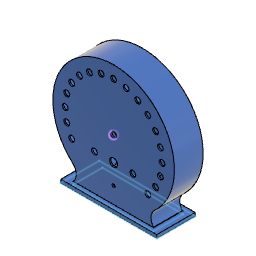
Minutka (Autodesk Fusion 360 design; units mm, degrees)
Autodesk Fusion 360 part; units mm, degrees
sketch "Sketch1" plane through (0, 0, 0) normal (0, 1, 0) x (1, 0, 0)
  circle A0 centre (0, 0) radius 35.5
  circle A1 centre (0, 0) radius 37
  circle A2 centre (0, 0) radius 38
  line L0 (-25, 37.5) -> (25, 37.5)
  line L1 (25, 37.5) -> (25, 39.5)
  line L2 (25, 39.5) -> (-25, 39.5)
  line L3 (-25, 39.5) -> (-25, 37.5)
  arc A3 (-25.5469, 28.131) -> (-25, 37.5) centre (-30.0546, 33.0946) ccw
  arc A4 (25, 37.5) -> (25.5469, 28.131) centre (30.0546, 33.0946) ccw
  dimension "d1" = 71
  dimension "d2" = 74
  dimension "d3" = 76
  dimension "d4" = 50
  dimension "d5" = 2
  dimension "d6" = 37.5
  dimension "d7" = 25
  constraint coincident A0.centre A1.centre
  constraint concentric A1 A2
  constraint horizontal L0
  constraint vertical L1
  constraint horizontal L2
  constraint vertical L3
  constraint tangent A2 A3
  constraint coincident A2 A3.start
  measures "d1" diameter of A0
  measures "d2" diameter of A1
  measures "d3" diameter of A2
  measures "d4" distance of L0.start L0.end
  measures "d5" distance of L0.start L2.end
  measures "d6" vertical distance of A0.centre L0.end
  measures "d7" horizontal distance of A0.centre L0.end
extrude "Extrude1" add sketch "Sketch1" along normal blind 18 contours A2 L0 | A2 L0 A4 | A2 L0 A3 | A2 L0 | A2 L0 L1 L2 L3 makes body 1
extrude "Extrude2" add sketch "Sketch1" along normal blind 17.2 contours A1 bodies 1
extrude "Extrude3" add sketch "Sketch1" along normal blind 0.8 contours A0 bodies 1
sketch "Sketch2" plane through (0, 17.2, 0) normal (0, 1, 0) x (-1, 0, 0)
  circle A0 centre (0, 0) radius 35.5
  circle A1 centre (0, 0) radius 37
  line L0 (-1.5, 38.5) -> (1.5, 38.5)
  line L1 (1.5, 38.5) -> (1.5, 35)
  line L2 (1.5, 35) -> (-1.5, 35)
  line L3 (-1.5, 35) -> (-1.5, 38.5)
  line L4 (-1.5, -42.5) -> (1.5, -42.5)
  line L5 (1.5, -42.5) -> (1.5, -34.5)
  line L6 (1.5, -34.5) -> (-1.5, -34.5)
  line L7 (-1.5, -34.5) -> (-1.5, -42.5)
  constraint horizontal L0
  constraint vertical L1
  constraint horizontal L2
  constraint vertical L3
  constraint horizontal L4
  constraint vertical L5
  constraint horizontal L6
  constraint vertical L7
extrude "Extrude4" cut sketch "Sketch2" against normal blind 1 contours A0 A1 L1 L3 | A0 A1 L5 L7 bodies 1
sketch "Sketch3" plane through (0, 0, 0) normal (0, 1, 0) x (1, 0, 0)
  circle A0 centre (-30.3, 0) radius 1.8
  circle A1 centre (-29.2676, 7.8422) radius 1.8
  circle A2 centre (-26.2406, 15.15) radius 1.8
  circle A3 centre (-29.2676, -7.8422) radius 1.8
  circle A4 centre (-26.2406, -15.15) radius 1.8
  circle A5 centre (-21.4253, -21.4253) radius 1.8
  circle A6 centre (-15.15, -26.2406) radius 1.8
  circle A7 centre (-7.8422, -29.2676) radius 1.8
  circle A8 centre (0, -30.3) radius 1.8
  circle A9 centre (7.8422, -29.2676) radius 1.8
  circle A10 centre (15.15, -26.2406) radius 1.8
  circle A11 centre (21.4253, -21.4253) radius 1.8
  circle A12 centre (26.2406, -15.15) radius 1.8
  circle A13 centre (29.2676, -7.8422) radius 1.8
  circle A14 centre (30.3, 0) radius 1.8
  circle A15 centre (29.2676, 7.8422) radius 1.8
  circle A16 centre (26.2406, 15.15) radius 1.8
  circle A17 centre (21.4253, 21.4253) radius 1.8
  circle A18 centre (0, 0) radius 1.8
  circle A19 centre (0, 27.5) radius 1
  circle A20 centre (0, 15) radius 2.5
  circle A21 centre (-12, 15) radius 1.8
  circle A22 centre (12, 15) radius 1.8
  dimension "d16" = 3.6
  dimension "d17" = 30.3
  dimension "d19" = -30
  dimension "d21" = 225
  dimension "d22" = 3.6
  dimension "d23" = 2
  dimension "d24" = 27.5
  dimension "d25" = 5
  dimension "d26" = 15
  dimension "d27" = 3.6
  dimension "d28" = 12
  dimension "d29" = 3.6
  dimension "d30" = 12
  constraint coincident A18.centre origin
  measures "d16" diameter of A0
  measures "d17" distance of A18.centre A0.centre
  measures "d22" diameter of A18
  measures "d23" diameter of A19
  measures "d24" distance of A18.centre A19.centre
  measures "d25" diameter of A20
  measures "d26" distance of A18.centre A20.centre
  measures "d27" diameter of A21
  measures "d28" distance of A20.centre A21.centre
  measures "d29" diameter of A22
  measures "d30" distance of A20.centre A22.centre
extrude "Extrude5" cut sketch "Sketch3" along normal blind 0.8 bodies 1
sketch "Sketch4" plane through (0, 0, 0) normal (0, -1, 0) x (1, 0, 0)
  circle A0 centre (12, -15) radius 1.8
  circle A1 centre (26.2406, -15.15) radius 1.8
  circle A2 centre (26.2406, 15.15) radius 1.8
  circle A3 centre (0, 30.3) radius 1.8
  circle A4 centre (-26.2406, 15.15) radius 1.8
  circle A5 centre (-26.2406, -15.15) radius 1.8
  circle A6 centre (-29.2676, 7.8422) radius 1.8
  circle A7 centre (-7.8422, 29.2676) radius 1.8
  circle A8 centre (21.4253, 21.4253) radius 1.8
  circle A9 centre (29.2676, -7.8422) radius 1.8
  circle A10 centre (0, -15) radius 2.5
  circle A11 centre (-12, -15) radius 1.8
  circle A12 centre (21.4253, -21.4253) radius 1.8
  circle A13 centre (29.2676, 7.8422) radius 1.8
  circle A14 centre (7.8422, 29.2676) radius 1.8
  circle A15 centre (-21.4253, 21.4253) radius 1.8
  circle A16 centre (-29.2676, -7.8422) radius 1.8
  circle A17 centre (-30.3, 0) radius 1.8
  circle A18 centre (-15.15, 26.2406) radius 1.8
  circle A19 centre (15.15, 26.2406) radius 1.8
  circle A20 centre (30.3, 0) radius 1.8
  circle A21 centre (0, -27.5) radius 1
  circle A22 centre (0, 0) radius 1.8
  line L0 (-25, -39.5) -> (25, -39.5)
  line L1 (25, -39.5) -> (25, -37.5)
  arc A23 (25.5469, -28.131) -> (25, -37.5) centre (30.0546, -33.0946) ccw
  arc A24 (25.5469, -28.131) -> (-25.5469, -28.131) centre (0, 0) ccw
  arc A25 (-25, -37.5) -> (-25.5469, -28.131) centre (-30.0546, -33.0946) ccw
  line L2 (-25, -37.5) -> (-25, -39.5)
  circle A26 centre (-10, -22.5) radius 3
  circle A27 centre (10, -22.5) radius 3
  circle A28 centre (0, 23) radius 3
  circle A29 centre (8, 23) radius 3
  dimension "d33" = 6
  dimension "d34" = 22.5
  dimension "d35" = 10
  dimension "d36" = 6
  dimension "d37" = 10
  dimension "d38" = 22.5
  dimension "d39" = 6
  dimension "d40" = 23
  dimension "d41" = 6
  dimension "d42" = 8
  measures "d33" diameter of A26
  measures "d34" vertical distance of A22.centre A26.centre
  measures "d35" horizontal distance of A22.centre A26.centre
  measures "d36" diameter of A27
  measures "d37" horizontal distance of A22.centre A27.centre
  measures "d38" vertical distance of A22.centre A27.centre
  measures "d39" diameter of A28
  measures "d40" distance of A22.centre A28.centre
  measures "d41" diameter of A29
  measures "d42" distance of A28.centre A29.centre
extrude "Extrude6" add sketch "Sketch4" against normal blind 8.8 contours A26 | A29 bodies 1
extrude "Extrude7" add sketch "Sketch4" against normal blind 17.2 contours A27 | A28 bodies 1
sketch "Sketch5" plane through (0, 8.8, 0) normal (0, 1, 0) x (-1, 0, 0)
  circle A0 centre (-8, 23) radius 3
  circle A1 centre (-8, 23) radius 1.25
  circle A2 centre (10, -22.5) radius 1.25
  dimension "d47" = 2.5
  dimension "d48" = 2.5
  constraint concentric A0 A1
  measures "d47" diameter of A1
  measures "d48" diameter of A2
extrude "Extrude8" cut sketch "Sketch5" against normal blind 7 contours A1 | A2 bodies 1
sketch "Sketch6" plane through (0, 17.2, 0) normal (0, 1, 0) x (-1, 0, 0)
  circle A0 centre (0, 23) radius 3
  circle A1 centre (0, 23) radius 1.25
  circle A2 centre (-10, -22.5) radius 1.25
  dimension "d51" = 2.5
  dimension "d52" = 2.5
  constraint concentric A0 A1
  measures "d51" diameter of A1
  measures "d52" diameter of A2
sketch "Sketch7" plane through (0, 0.8, 0) normal (0, 1, 0) x (-1, 0, 0)
  circle A0 centre (-10, -22.5) radius 3
  circle A1 centre (0, 23) radius 3
  circle A2 centre (10, -22.5) radius 3
  circle A3 centre (-8, 23) radius 3
  circle A4 centre (-12, -15) radius 1.8
  circle A5 centre (-26.2406, -15.15) radius 1.8
  circle A6 centre (-26.2406, 15.15) radius 1.8
  circle A7 centre (0, 30.3) radius 1.8
  circle A8 centre (26.2406, 15.15) radius 1.8
  circle A9 centre (26.2406, -15.15) radius 1.8
  circle A10 centre (29.2676, 7.8422) radius 1.8
  circle A11 centre (7.8422, 29.2676) radius 1.8
  circle A12 centre (-21.4253, 21.4253) radius 1.8
  circle A13 centre (-29.2676, -7.8422) radius 1.8
  circle A14 centre (0, -15) radius 2.5
  circle A15 centre (12, -15) radius 1.8
  circle A16 centre (-21.4253, -21.4253) radius 1.8
  circle A17 centre (-29.2676, 7.8422) radius 1.8
  circle A18 centre (-7.8422, 29.2676) radius 1.8
  circle A19 centre (21.4253, 21.4253) radius 1.8
  circle A20 centre (29.2676, -7.8422) radius 1.8
  circle A21 centre (30.3, 0) radius 1.8
  circle A22 centre (15.15, 26.2406) radius 1.8
  circle A23 centre (-15.15, 26.2406) radius 1.8
  circle A24 centre (-30.3, 0) radius 1.8
  circle A25 centre (0, -27.5) radius 1
  circle A26 centre (0, 0) radius 1.8
  circle A27 centre (0, 0) radius 35.5
extrude "Extrude9" cut sketch "Sketch6" against normal blind 12 contours A1 | A2 bodies 1
sketch "Sketch8" plane through (0, 17.2, 0) normal (0, 1, 0) x (-1, 0, 0)
  line L0 (-1.5, 35.4683) -> (-1.5, 36.9696)
  arc A0 (-1.5, 36.9696) -> (-1.5, -36.9696) centre (0, 0) ccw
  line L1 (-1.5, -36.9696) -> (-1.5, -35.4683)
  arc A1 (-1.5, 35.4683) -> (-1.5, -35.4683) centre (0, 0) ccw
  circle A2 centre (0, 0) radius 36.5
  line L2 (-1.25, 38.5) -> (1.25, 38.5)
  line L3 (1.25, 38.5) -> (1.25, 34.7673)
  line L4 (1.25, 34.7673) -> (-1.25, 34.7673)
  line L5 (-1.25, 34.7673) -> (-1.25, 38.5)
  circle A3 centre (0, 0) radius 37
  line L6 (-1.25, -34) -> (1.25, -34)
  line L7 (1.25, -34) -> (1.25, -38.157)
  line L8 (1.25, -38.157) -> (-1.25, -38.157)
  line L9 (-1.25, -38.157) -> (-1.25, -34)
  circle A4 centre (-10, -22.5) radius 1.5
  circle A5 centre (0, 23) radius 1.5
  dimension "d55" = 73
  dimension "d56" = 2.5
  dimension "d57" = 1.25
  dimension "d58" = 2.5
  dimension "d59" = 1.25
  dimension "d60" = 3
  dimension "d61" = 3
  constraint coincident A0.centre A1.centre
  constraint horizontal L2
  constraint vertical L3
  constraint horizontal L4
  constraint vertical L5
  constraint horizontal L6
  constraint vertical L7
  constraint horizontal L8
  constraint vertical L9
  measures "d55" diameter of A2
  measures "d56" distance of L2.start L2.end
  measures "d57" horizontal distance of L2.start A0.centre
  measures "d58" distance of L6.start L6.end
  measures "d59" horizontal distance of A0.centre L6.start
  measures "d60" diameter of A4
  measures "d61" diameter of A5
extrude "Extrude10" add sketch "Sketch8" along normal blind 0.8 separate body contours L0 L1 A1 A2 | L0 L1 A1 A2 L3 L4 L5 L6 L7 L9 | A2 L3 L4 L5 | A2 L6 L7 L9 makes body 2
extrude "Extrude11" add sketch "Sketch8" against normal blind 0.5 contours A2 L3 L4 L5 | A2 L6 L7 L9 bodies 2
sketch "Sketch9" plane through (0, 0, 0) normal (0, 0, 1) x (1, 0, 0)
  line L0 (-30, 21, -39.5) -> (30, 21, -39.5)
  line L1 (30, 21, -39.5) -> (30, -3, -39.5)
  line L2 (30, -3, -39.5) -> (-30, -3, -39.5)
  line L3 (-30, -3, -39.5) -> (-30, 21, -39.5)
  line L4 (-25.25, 18.25, -39.5) -> (25.25, 18.25, -39.5)
  line L5 (25.25, 18.25, -39.5) -> (25.25, -0.25, -39.5)
  line L6 (25.25, -0.25, -39.5) -> (-25.25, -0.25, -39.5)
  line L7 (-25.25, -0.25, -39.5) -> (-25.25, 18.25, -39.5)
  point P0 (0, 0)
  dimension "d66" = 60
  dimension "d67" = 24
  dimension "d70" = 50.5
  dimension "d71" = 18.5
extrude "Extrude14" add sketch "Sketch9" along normal blind 2 separate body contours L0 L1 L2 L3 in plane through (0, 0, -39.5) normal (0, 0, 1) makes body 3
extrude "Extrude15" add sketch "Sketch9" along normal blind 0.5 contours L4 L5 L6 L7 in plane through (0, 0, -39.5) normal (0, 0, 1) bodies 3
